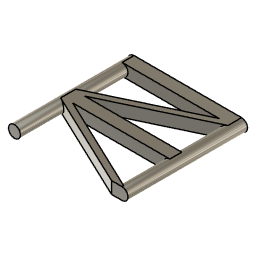
RollerCoasterRail (Autodesk Fusion 360 design; units mm, degrees)
Autodesk Fusion 360 part; units mm, degrees
sketch "スケッチ1" plane through (0, 0, 0) normal (0, 0, 1) x (1, 0, 0)
  line L0 (-500, 0) -> (500, 0)
  line L1 (500, 0) -> (500, -1000)
  line L2 (-500, -1000) -> (-500, 0)
  line L3 (-400, -100) -> (362.4762, -100)
  line L4 (400, -137.5238) -> (400, -500)
  line L5 (400, -500) -> (-362.4762, -500)
  line L6 (-400, -462.4762) -> (-400, -100)
  line L7 (-362.4762, -600) -> (400, -600)
  line L8 (400, -600) -> (400, -962.4762)
  line L9 (400, -1000) -> (362.4762, -1000)
  line L10 (-400, -1000) -> (-400, -637.5238)
  line L11 (-400, -462.4762) -> (362.4762, -100)
  line L12 (400, -137.5238) -> (-362.4762, -500)
  line L13 (-362.4762, -600) -> (400, -962.4762)
  line L14 (362.4762, -1000) -> (-400, -637.5238)
  line L15 (500, -1000) -> (362.4762, -1000)
  line L16 (-400, -1000) -> (-500, -1000)
  line L17 (-400, -462.4762) -> (-400, -500) construction
  line L18 (-400, -500) -> (-362.4762, -500) construction
  line L19 (-362.4762, -600) -> (-400, -600) construction
  line L20 (-400, -600) -> (-400, -637.5238) construction
  line L21 (362.4762, -100) -> (400, -100) construction
  line L22 (400, -100) -> (400, -137.5238) construction
  line L23 (400, -962.4762) -> (400, -1000) construction
  line L24 (-400, -1000) -> (362.4762, -1000) construction
  dimension "d5" = 400
  dimension "d6" = 800
  dimension "d7" = 100
  dimension "d8" = 100
  dimension "d9" = 100
  dimension "d10" = 100
  dimension "d11" = 400
  dimension "d12" = 50
  dimension "d13" = 50
  constraint horizontal L0
  constraint vertical L1
  constraint horizontal L15
  constraint vertical L2
  constraint horizontal L3
  constraint vertical L4
  constraint horizontal L5
  constraint vertical L6
  constraint horizontal L7
  constraint vertical L8
  constraint horizontal L9
  constraint vertical L10
  constraint coincident L9.start L15
  constraint parallel L11 L12
  constraint parallel L13 L14
  constraint collinear L15 L16
  constraint perpendicular L5 L17
  constraint perpendicular L17 L18
  constraint parallel L7 L19
  constraint perpendicular L19 L20
  constraint perpendicular L1 L21
  constraint perpendicular L21 L22
  constraint perpendicular L9 L23
  constraint collinear L6 L10
  constraint collinear L4 L8
  constraint equal L17 L18
  constraint equal L19 L20
  constraint equal L21 L22
  constraint equal L9 L23
  constraint midpoint origin L0
  measures "d5" distance of L3.start L17.end
  measures "d6" distance of L3.start L21.end
  measures "d7" distance of L2 L3.start
  measures "d8" distance of L1 L21.end
  measures "d9" distance of L0 L3.start
  measures "d10" distance of L17.end L19.end
  measures "d11" distance of L10.start L19.end
  measures "d12" distance of L11 L12
  measures "d13" distance of L13 L14
extrude "押し出し1" add sketch "スケッチ1" along normal blind 100
fillet "フィレット1" radius 50 1 edges at (-500, -500, 100)
fillet "フィレット2" radius 50 1 edges at (-400, -281.2381, 100)
fillet "フィレット3" radius 50 1 edges at (-400, -818.7619, 100)
fillet "フィレット4" radius 50 3 edges at (400, -318.7619, 100) (400, -781.2381, 100) (500, -500, 100)
fillet "フィレット5" radius 50 6 edges at (-500, -500, 0) (-400, -818.7619, 0) (-400, -281.2381, 0) (400, -318.7619, 0) (400, -781.2381, 0) (500, -500, 0)
